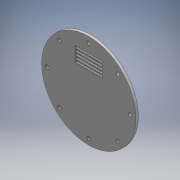
# Autodesk Inventor part: Baseplate
Saved by Autodesk Inventor 2016 (Build 200138000, 138)
## iProperties
Created: 2016-03-21
Part Number: Baseplate
Material: Generic
Document SubType Name: Modeling
Designer: s_sud
Density: 1 g/cm^3
Appearance: Default
Author: s_sud
Autodesk Inventor part; units mm, degrees
ref_plane "YZ Plane" through (0, 0, 0) normal (1, 0, 0) x (0, 1, 0)
ref_plane "XZ Plane" through (0, 0, 0) normal (0, 1, 0) x (-1, 0, 0)
ref_plane "XY Plane" through (0, 0, 0) normal (0, 0, 1) x (1, 0, 0)
sketch "Sketch1" plane through (0, 0, 0) normal (0, 1, 0) x (-1, 0, 0)
  circle A0 centre (0, 0) radius 75
  circle A1 centre (0, 65.8304) radius 2.8396
  circle A2 centre (-46.5491, 46.5491) radius 2.8396
  circle A3 centre (-65.8304, 0) radius 2.8396
  circle A4 centre (-46.5491, -46.5491) radius 2.8396
  circle A5 centre (0, -65.8304) radius 2.8396
  circle A6 centre (46.5491, -46.5491) radius 2.8396
  circle A7 centre (65.8304, 0) radius 2.8396
  circle A8 centre (46.5491, 46.5491) radius 2.8396
  line L0 (-21.1442, 51.6217) -> (21.1442, 51.6217)
  line L1 (21.1442, 51.6217) -> (21.1442, 48.6217)
  line L2 (21.1442, 48.6217) -> (-21.1442, 48.6217)
  line L3 (-21.1442, 48.6217) -> (-21.1442, 51.6217)
  line L4 (-21.1442, 51.6217) -> (21.1442, 48.6217) construction
  line L5 (21.1442, 51.6217) -> (-21.1442, 48.6217) construction
  line L6 (-21.1442, 46.6217) -> (21.1442, 46.6217)
  line L7 (21.1442, 46.6217) -> (21.1442, 43.6217)
  line L8 (21.1442, 43.6217) -> (-21.1442, 43.6217)
  line L9 (-21.1442, 43.6217) -> (-21.1442, 46.6217)
  line L10 (-21.1442, 46.6217) -> (21.1442, 43.6217) construction
  line L11 (21.1442, 46.6217) -> (-21.1442, 43.6217) construction
  line L12 (-21.1442, 41.6217) -> (21.1442, 41.6217)
  line L13 (21.1442, 41.6217) -> (21.1442, 38.6217)
  line L14 (21.1442, 38.6217) -> (-21.1442, 38.6217)
  line L15 (-21.1442, 38.6217) -> (-21.1442, 41.6217)
  line L16 (-21.1442, 41.6217) -> (21.1442, 38.6217) construction
  line L17 (21.1442, 41.6217) -> (-21.1442, 38.6217) construction
  line L18 (-21.1442, 36.6217) -> (21.1442, 36.6217)
  line L19 (21.1442, 33.6217) -> (-21.1442, 33.6217)
  line L20 (-21.1442, 33.6217) -> (-21.1442, 36.6217)
  line L21 (-21.1442, 36.6217) -> (21.1442, 33.6217) construction
  line L22 (21.1442, 36.6217) -> (-21.1442, 33.6217) construction
  line L23 (-21.1442, 31.6217) -> (21.1442, 31.6217)
  line L24 (21.1442, 28.6217) -> (-21.1442, 28.6217)
  line L25 (-21.1442, 28.6217) -> (-21.1442, 31.6217)
  line L26 (-21.1442, 31.6217) -> (21.1442, 28.6217) construction
  line L27 (21.1442, 31.6217) -> (-21.1442, 28.6217) construction
  line L28 (21.1442, 36.6217) -> (21.1442, 33.6217)
  line L29 (21.1442, 31.6217) -> (21.1442, 28.6217)
  point P0 (0, 50.1217)
  point P1 (0, 45.1217)
  point P2 (0, 40.1217)
  point P3 (0, 35.1217)
  point P4 (0, 30.1217)
  dimension "d0" = 150
  dimension "d3" = 360
  dimension "d5" = 3
  dimension "d6" = 3
  dimension "d7" = 3
  dimension "d8" = 2
  dimension "d9" = 2
  dimension "d12" = 3
  dimension "d15" = 3
  dimension "d16" = 2
  dimension "d17" = 2
  constraints: 60 end point, 10 midpoint, 9 centre point, 9 equal length, 5 horizontal, 3 perpendicular, 1 coincident, 1 point on line, 1 vertical, 17 other
  measures "d0" diameter of A0
  measures "d5" distance of L12.end L13.end
  measures "d6" distance of L6.end L7.end
  measures "d7" distance of L0.end L1.end
  measures "d8" distance between parallel lines of L2 L6
  measures "d9" distance between parallel lines of L8 L12
  measures "d12" distance of L18.end L19.start
  measures "d15" distance of L23.end L24.start
  measures "d16" distance between parallel lines of L14 L18
  measures "d17" distance between parallel lines of L19 L23
extrude "Extrusion1" add sketch "Sketch1" along normal blind 4
sketch "Sketch2" plane through (0, 4, 0) normal (0, 1, 0) x (1, 0, 0)
  point P0 (0, 0)
body "Solid1"
